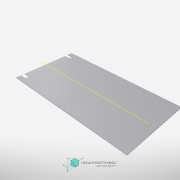
# Autodesk Inventor part: baseplate-alu
Saved by Autodesk Inventor 2016 (Build 200138000, 138)
## iProperties
Created: 2015-05-03
Part Number: baseplate-alu
Material: Aluminum 6061
Document SubType Name: Modeling
Designer: ax
Mass: 2363 g
Surface Area: 5922.43 cm^2
Volume: 875.186 cm^3
Density: 2.7 g/cm^3
Appearance: Aluminum - Flat
Author: ax
Autodesk Inventor part; units mm, degrees
ref_plane "YZ Plane" through (0, 0, 0) normal (1, 0, 0) x (0, 1, 0)
ref_plane "XZ Plane" through (0, 0, 0) normal (0, 1, 0) x (-1, 0, 0)
ref_plane "XY Plane" through (0, 0, 0) normal (0, 0, 1) x (1, 0, 0)
sketch "Sketch1" plane through (0, 0, 0) normal (0, 0, 1) x (1, 0, 0)
  line L0 (0, 0) -> (758, 0)
  line L1 (758, 0) -> (758, 400)
  line L2 (758, 400) -> (0, 400)
  line L3 (0, 400) -> (0, 0)
  dimension "d0" = 758
  dimension "d1" = 400
  constraints: 8 end point, 2 parallel, 1 horizontal, 1 perpendicular
  measures "d0" distance of L2.end L1.end
  measures "d1" distance of L1.end L0.end
extrude "Extrusion1" add sketch "Sketch1" along normal blind 3
sketch "Sketch2" plane through (0, 0, 0) normal (0, 0, -1) x (-1, 0, 0)
  line L0 (0, 0) -> (-758, 0) construction
  line L1 (0, 0) -> (-42, 0) construction
  line L2 (-42, 0) -> (-42, 32) construction
  line L3 (-42, 32) -> (0, 32) construction
  line L4 (0, 32) -> (0, 0) construction
  line L5 (0, 0) -> (-42, 0) construction
  line L6 (-42, 0) -> (-42, 54) construction
  line L7 (-42, 54) -> (0, 54) construction
  line L8 (0, 54) -> (0, 0) construction
  line L9 (-36, 32) -> (0, 32)
  line L10 (0, 32) -> (0, 54)
  line L11 (0, 54) -> (-36, 54)
  line L12 (-42, 48) -> (-42, 38)
  arc A0 (-42, 38) -> (-36, 32) centre (-36, 38) ccw
  arc A1 (-36, 54) -> (-42, 48) centre (-36, 48) ccw
  dimension "d4" = 42
  dimension "d5" = 32
  dimension "d6" = 54
  dimension "d7" = 6
  constraints: 24 end point, 6 parallel, 4 point on circle, 4 tangent, 3 horizontal, 3 perpendicular, 3 point on line, 2 centre point, 1 equal radius
  measures "d4" distance of L2.end L3.end
  measures "d5" distance of L1.end L2.end
  measures "d6" distance of L5.end L6.end
  measures "d7" radius of A0
extrude "Extrusion2" cut sketch "Sketch2" against normal through all
sketch "Sketch3" plane through (0, 0, 0) normal (0, 0, -1) x (-1, 0, 0)
  line L0 (0, 0) -> (-758, 0) projected
  line L1 (0, 32) -> (0, 0) projected
  point P0 (-7.5, 13.5)
  point P1 (-32.5, 13.5)
  point P2 (-57.5, 13.5)
  point P3 (-82.5, 13.5)
  point P4 (-107.5, 13.5)
  point P5 (-132.5, 13.5)
  point P6 (-157.5, 13.5)
  point P7 (-182.5, 13.5)
  point P8 (-207.5, 13.5)
  point P9 (-232.5, 13.5)
  point P10 (-257.5, 13.5)
  point P11 (-282.5, 13.5)
  point P12 (-307.5, 13.5)
  point P13 (-332.5, 13.5)
  point P14 (-357.5, 13.5)
  point P15 (-382.5, 13.5)
  point P16 (-407.5, 13.5)
  point P17 (-432.5, 13.5)
  point P18 (-457.5, 13.5)
  point P19 (-482.5, 13.5)
  point P20 (-507.5, 13.5)
  point P21 (-532.5, 13.5)
  point P22 (-557.5, 13.5)
  point P23 (-582.5, 13.5)
  point P24 (-607.5, 13.5)
  point P25 (-632.5, 13.5)
  point P26 (-657.5, 13.5)
  dimension "d10" = 13.5
  dimension "d11" = 7.5
  dimension "d14" = 25
  constraints: 1 horizontal, 26 other
  measures "d10" distance from line of L0 point (-7.5, 13.5)
  measures "d11" distance from line of L1 point (-7.5, 13.5)
  measures "d14" distance of point (-7.5, 13.5) point (-32.5, 13.5)
hole "Hole1" at (32.5, 13.5, 0) at (57.5, 13.5, 0) at (82.5, 13.5, 0) at (107.5, 13.5, 0) at (132.5, 13.5, 0) at (157.5, 13.5, 0) at (182.5, 13.5, 0) at (207.5, 13.5, 0) at (232.5, 13.5, 0) at (282.5, 13.5, 0) at (307.5, 13.5, 0) at (332.5, 13.5, 0) at (357.5, 13.5, 0) at (382.5, 13.5, 0) at (407.5, 13.5, 0) at (432.5, 13.5, 0) at (457.5, 13.5, 0) at (482.5, 13.5, 0) at (507.5, 13.5, 0) at (532.5, 13.5, 0) at (557.5, 13.5, 0) at (582.5, 13.5, 0) at (607.5, 13.5, 0) at (632.5, 13.5, 0) at (657.5, 13.5, 0) at (257.5, 13.5, 0) at (7.5, 13.5, 0) direction (0, 0, 1) diameter 2.459 end through all thread size "M3x0.5" class "6H" standard "ISO Metric profile"
ref_plane "Work Plane1" through (0, 200, 0) normal (0, -1, 0) x (1, 0, 0)
sketch "Sketch4" plane through (0, 0, 0) normal (0, 0, -1) x (-1, 0, 0)
  line L0 (-758, 0) -> (-680, 0)
  line L1 (-680, 0) -> (-680, 60)
  line L2 (-680, 60) -> (-758, 60)
  line L3 (-758, 60) -> (-758, 0)
  point P0 (0, 0)
  dimension "d26" = 78
  dimension "d27" = 60
  constraints: 8 end point, 2 parallel, 1 horizontal, 1 perpendicular
  measures "d26" distance of L2.end L1.end
  measures "d27" distance of L1.end L0.end
extrude "Extrusion3" cut sketch "Sketch4" against normal through all
mirror "Mirror1" about plane through (0, 200, 0) normal (0, -1, 0) of "Hole1", "Extrusion2", "Extrusion3"
hole "Hole2" at (753, 335, 3) direction (0, 0, -1) diameter 4 end through all
pattern_linear "Rectangular Pattern1" count 3 spacing 135 along (0, -1, 0) of "Hole2"
body "Solid1"
